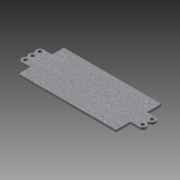
# Autodesk Inventor part: PowerPCB
Saved by Autodesk Inventor 2016 (Build 200138000, 138)
## iProperties
Created: 2015-06-09
Part Number: PowerPCB
Material: GFRC
Document SubType Name: Modeling
Designer: Yann
Density: 1.7 g/cm^3
Appearance: Flat - Polished Gray
Author: Yann
Autodesk Inventor part; units mm, degrees
ref_plane "YZ Plane" through (0, 0, 0) normal (1, 0, 0) x (0, 1, 0)
ref_plane "XZ Plane" through (0, 0, 0) normal (0, 1, 0) x (-1, 0, 0)
ref_plane "XY Plane" through (0, 0, 0) normal (0, 0, 1) x (1, 0, 0)
sketch "Sketch1" plane through (0, 0, 0) normal (0, 0, 1) x (1, 0, 0)
  line L0 (0, 44.1) -> (0, -44.1) construction
  line L1 (-3497.9632, 0) -> (3497.9632, 0) construction
  line L2 (0, -31.5) -> (-68, -31.5)
  line L3 (-68, -31.5) -> (-68, -18)
  line L4 (-68, -18) -> (-80, -18)
  line L5 (-85, 0) -> (-85, -22.0738) construction
  line L6 (-75, -22.5739) -> (-75, 22.5739) construction
  circle A0 centre (-80, -13) radius 2.5
  circle A1 centre (-80, 0) radius 2.5
  line L7 (-80, 0) -> (-80, -13) construction
  arc A2 (-81.8558, -8.3571) -> (-80, -18) centre (-80, -13) ccw
  arc A3 (-85, 0) -> (-81.8558, -4.6429) centre (-80, 0) ccw
  arc A4 (-81.8558, -8.3571) -> (-81.8558, -4.6429) centre (-82.5981, -6.5) ccw
  line L8 (0, 31.5) -> (-68, 31.5)
  line L9 (-68, 31.5) -> (-68, 18)
  line L10 (-68, 18) -> (-80, 18)
  line L11 (-85, 0) -> (-85, 22.0738) construction
  line L12 (-75, 22.5739) -> (-75, -22.5739) construction
  circle A5 centre (-80, 13) radius 2.5
  circle A6 centre (-80, 0) radius 2.5
  line L13 (-80, 0) -> (-80, 13) construction
  arc A7 (-80, 18) -> (-81.8558, 8.3571) centre (-80, 13) ccw
  arc A8 (-81.8558, 4.6429) -> (-85, 0) centre (-80, 0) ccw
  arc A9 (-81.8558, 4.6429) -> (-81.8558, 8.3571) centre (-82.5981, 6.5) ccw
  line L14 (3497.9632, 0) -> (-3497.9632, 0) construction
  line L15 (0, -31.5) -> (68, -31.5)
  line L16 (68, -31.5) -> (68, -11.5)
  line L17 (68, -11.5) -> (80, -11.5)
  line L18 (68, 11.5) -> (80, 11.5)
  line L19 (68, 31.5) -> (68, 11.5)
  line L20 (0, 31.5) -> (68, 31.5)
  line L21 (80, 11.5) -> (80, -11.5) construction
  circle A10 centre (80, -6.5) radius 2.5
  circle A11 centre (80, 6.5) radius 2.5
  line L22 (75, 22.5739) -> (75, -22.5739) construction
  line L23 (75, 22.5739) -> (75, -22.5739) construction
  arc A12 (80, -11.5) -> (81.8558, -1.8571) centre (80, -6.5) ccw
  arc A13 (81.8558, 1.8571) -> (80, 11.5) centre (80, 6.5) ccw
  arc A14 (81.8558, 1.8571) -> (81.8558, -1.8571) centre (82.5981, 0) ccw
  point P0 (0, 0)
  dimension "d0" = 31.5
  dimension "d2" = 7
  dimension "d4" = 5
  dimension "d5" = 5
  dimension "d6" = 5
  dimension "d7" = 5
  dimension "d8" = 13
  dimension "d9" = 5
  dimension "d10" = 2
  dimension "d11" = 2.5
  dimension "d12" = 5
  dimension "d13" = 2.5
  dimension "d14" = 5
  dimension "d15" = 13
  dimension "d16" = 2
  constraints: 36 end point, 18 point on circle, 17 symmetric about line, 15 centre point, 6 coincident, 6 point on line, 4 tangent, 4 vertical, 2 horizontal, 2 perpendicular, 7 other
  measures "d0" distance between parallel lines of L2 L1
  measures "d2" distance between parallel lines of L3 L6
  measures "d4" diameter of A0
  measures "d5" diameter of A1
  measures "d6" distance from line of L5 L7.start
  measures "d7" distance from line of L7.end L5
  measures "d8" distance of L7.start L7.end
  measures "d9" distance from line of L4 L7.end
  measures "d10" radius of A4
  measures "d11" distance edge to line of A0 L6
  measures "d12" diameter of A10
  measures "d13" distance edge to line of A10 L22
  measures "d14" distance from line of L17 A10.centre
  measures "d15" distance of A10.centre A11.centre
  measures "d16" radius of A14
extrude "Extrusion1" add sketch "Sketch1" along normal blind 3
equation "\"d0\" = 0.5 * PowerPCB_Width"
equation "\"d2\" = Interface_Thickness"
equation "\"d7\" = d6"
equation "\"d12\" = d4"
equation "\"d13\" = d11"
equation "\"d14\" = d9"
equation "\"d17\" = PowerPCB_Thickness"
equation "\"Heatsink_Thickness\" = 5"
equation "\"Heatsink_Width\" = 65"
equation "\"Cover_Thickness\" = 2"
equation "\"PowerPCB_Minus_Height\" = 1.2"
equation "\"PowerPCB_Width\" = 63"
equation "\"Interface_Thickness\" = 7"
equation "\"PowerPCB_Thickness\" = 3"
equation "\"PowerPCB_Plus_Height\" = 8"
equation "\"LogicPCB_Width\" = 55"
equation "\"LogicPCB_Thickness\" = 2"
equation "\"LogicPCB_Plus_Height\" = 8"
equation "\"HostPCB_Thickness\" = 1.2"
equation "\"HostPCB_Plus_Height\" = 8"
body "Solid1"
